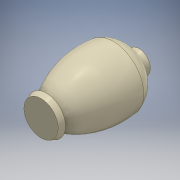
# Autodesk Inventor part: 도자기
Saved by Autodesk Inventor 2016 (Build 200138000, 138)
## iProperties
Created: 2024-03-15
Part Number: 도자기
Material: 자기, 리넨
Document SubType Name: Modeling
Designer: pc
Density: 3.4 g/cm^3
Appearance: 화창한 날
Author: pc
Autodesk Inventor part; units mm, degrees
ref_plane "YZ Plane" through (0, 0, 0) normal (1, 0, 0) x (0, 1, 0)
ref_plane "XZ Plane" through (0, 0, 0) normal (0, 1, 0) x (-1, 0, 0)
ref_plane "XY Plane" through (0, 0, 0) normal (0, 0, 1) x (1, 0, 0)
sketch "스케치1" plane through (0, 0, 0) normal (0, 0, 1) x (1, 0, 0)
  line L0 (-0.0017, 94.0937) -> (-21.0798, 94.0937)
  arc A0 (-17.8212, 81.9159) -> (-55.9018, 47.0217) centre (-5.845, 30.6199) ccw
  arc A1 (-55.9018, 47.0217) -> (-22.3451, -76.2024) centre (104.7389, 24.5866) ccw
  line L1 (-22.3451, -76.2024) -> (-35.2784, -76.2024)
  line L2 (-35.2784, -76.2024) -> (-31.5224, -85.9063)
  line L3 (-31.5224, -85.9063) -> (-0.0017, -85.9063)
  line L4 (-0.0017, -85.9063) -> (-0.0017, 94.0937)
  line L5 (-21.0798, 94.0937) -> (-17.0393, 81.7756)
  line L6 (-17.0393, 81.7756) -> (-17.8212, 81.9159)
  arc A2 (-55.9018, 47.0217) -> (-86.3474, 26.4808) centre (-69.7124, 34.6582) ccw
  arc A3 (-86.3474, 26.4808) -> (-55.905, 2.1748) centre (-45.3202, 46.6488) ccw
  point P0 (0, 0)
  dimension "d0" = 180
  constraints: 14 end point, 9 point on circle, 4 centre point, 2 horizontal, 1 parallel, 1 perpendicular, 1 tangent
  measures "d0" distance of L3.end L0.start
revolve "회전1" add sketch "스케치1" angle 360 about axis through (-0.0017, -85.9063, 0) along (0, 1, 0) contours L4 L3 L2 L1 A1 A0 L6 L5 L0
sketch "스케치2" plane through (-0.0017, 94.0937, 0) normal (0, 1, 0) x (1, 0, 0)
  point P0 (0.0017, 0)
shell "쉘1" thickness 2 removed faces 1 at (4.7197, 94.0937, 2.478)
sketch "스케치3" plane through (-0.0017, 94.0937, 0) normal (0, 1, 0) x (1, 0, 0)
  point P0 (0.0017, 0)
